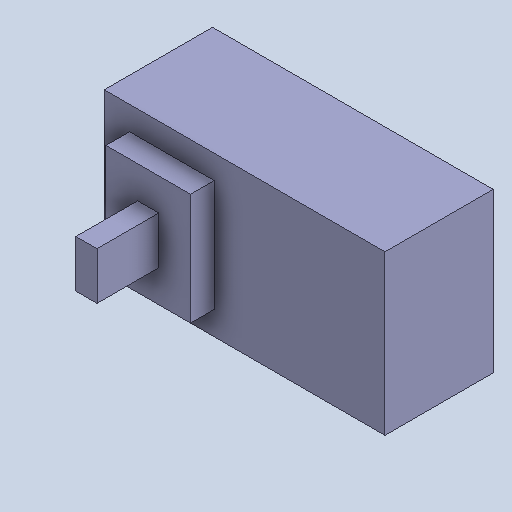
# Autodesk Inventor part: poeAdapter
Saved by Autodesk Inventor 2023 (Build 270158030, 158C)
## iProperties
Created: 2021-08-20
Part Number: poeAdapter
Material: PC/ABS Plastic
Document SubType Name: Modeling
Designer: robst
Density: 0.357273 g/cm^3
Appearance: Slate Blue
Author: robst
Autodesk Inventor part; units mm, degrees
ref_plane "YZ Plane" through (0, 0, 0) normal (1, 0, 0) x (0, 1, 0)
ref_plane "XZ Plane" through (0, 0, 0) normal (0, 1, 0) x (-1, 0, 0)
ref_plane "XY Plane" through (0, 0, 0) normal (0, 0, 1) x (1, 0, 0)
sketch "Sketch8" plane through (0, 0, 0) normal (0, 0, 1) x (1, 0, 0)
  line L0 (-41.5, -23.5) -> (41.5, -23.5)
  line L1 (41.5, -23.5) -> (41.5, 23.5)
  line L2 (41.5, 23.5) -> (-41.5, 23.5)
  line L3 (-41.5, 23.5) -> (-41.5, -23.5)
  line L4 (-41.5, -23.5) -> (41.5, 23.5) construction
  line L5 (41.5, -23.5) -> (-41.5, 23.5) construction
  point P0 (0, 0)
  dimension "d31" = 47
  dimension "d32" = 83
  constraints: 12 end point, 2 midpoint, 2 parallel, 1 horizontal, 1 perpendicular
  measures "d31" distance of L0.end L1.end
  measures "d32" distance of L1.end L2.end
extrude "Extrusion6" add sketch "Sketch8" against normal blind 32
sketch "Sketch9" plane through (0, 0, 0) normal (0, 0, 1) x (1, 0, 0)
  line L0 (-41.5, -23.5) -> (-41.5, 23.5) construction
  line L1 (-41.5, 0) -> (41.5, 0) construction
  line L2 (41.5, 23.5) -> (41.5, -23.5) construction
  line L3 (-34, -16.5) -> (-9, -16.5)
  line L4 (-9, -16.5) -> (-9, 16.5)
  line L5 (-9, 16.5) -> (-34, 16.5)
  line L6 (-34, 16.5) -> (-34, -16.5)
  line L7 (-34, -16.5) -> (-9, 16.5) construction
  line L8 (-9, -16.5) -> (-34, 16.5) construction
  point P0 (0, 0)
  point P1 (-21.5, 0)
  point P2 (-21.5, 0)
  dimension "d35" = 20
  dimension "d36" = 25
  dimension "d37" = 33
  constraints: 14 end point, 5 midpoint, 2 parallel, 1 perpendicular, 1 point on line
  measures "d35" distance from line of point (-21.5, 0) L0
  measures "d36" distance of L4.end L5.end
  measures "d37" distance of L5.end L3.start
extrude "Extrusion7" add sketch "Sketch9" along normal blind 7
sketch "Sketch10" plane through (0, 0, 7) normal (0, 0, 1) x (1, 0, 0)
  line L0 (-34, -16.5) -> (-34, 16.5) construction
  line L1 (-34, 0) -> (-9, 0) construction
  line L2 (-9, 16.5) -> (-9, -16.5) construction
  line L3 (-24.625, -7) -> (-18.375, -7)
  line L4 (-18.375, -7) -> (-18.375, 7)
  line L5 (-18.375, 7) -> (-24.625, 7)
  line L6 (-24.625, 7) -> (-24.625, -7)
  line L7 (-24.625, -7) -> (-18.375, 7) construction
  line L8 (-18.375, -7) -> (-24.625, 7) construction
  line L9 (-41.5, 23.5) -> (-41.5, -23.5) projected
  point P0 (0, 0)
  point P1 (-21.5, 0)
  point P2 (-21.5, 0)
  dimension "d40" = 20
  dimension "d41" = 14
  dimension "d42" = 6.25
  constraints: 14 end point, 6 midpoint, 2 parallel, 1 perpendicular
  measures "d40" distance from line of point (-21.5, 0) L9
  measures "d41" distance of L5.end L3.start
  measures "d42" distance of L3.start L3.end
extrude "Extrusion8" add sketch "Sketch10" along normal blind 18.28
equation "\"d31\" = poeWidth"
equation "\"d32\" = poeLength"
equation "\"d33\" = poeMajorDepth"
equation "\"d35\" = plugBaseCenterFromTop"
equation "\"d36\" = plugBaseLength"
equation "\"d37\" = plugBaseWidth"
equation "\"d38\" = plugBaseDepth"
equation "\"d40\" = plugCenterFromTop"
equation "\"d41\" = plugWidth"
equation "\"d42\" = plugLength"
equation "\"d43\" = plugDepth"
equation "\"poeLength\" = 83"
equation "\"poeWidth\" = 47"
equation "\"poeMajorDepth\" = 32"
equation "\"plugBaseWidth\" = 33"
equation "\"plugBaseLength\" = 25"
equation "\"plugBaseDepth\" = 7"
equation "\"plugBaseCenterFromTop\" = 20"
equation "\"plugWidth\" = 14"
equation "\"plugLength\" = 6.25"
equation "\"plugDepth\" = 18.28"
equation "\"plugCenterFromTop\" = 20"
body "Solid2"
